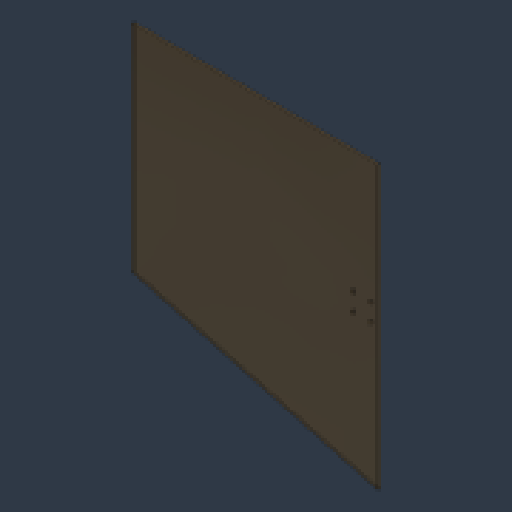
# Autodesk Inventor part: hopper_side_l
Saved by Autodesk Inventor 2024.3 (Build 283343000, 343)
## iProperties
Created: 2025-03-07
Part Number: hopper_side_l
Material: Polycarbonate, Smoke
Document SubType Name: Sheet Metal
Designer: marcu
Density: 1.2 g/cm^3
Sheet Metal Rule: Default
Appearance: Polycarbonate - Smoked
Author: marcu
Autodesk Inventor part; units mm, degrees
ref_plane "YZ Plane" through (0, 0, 0) normal (1, 0, 0) x (0, 1, 0)
ref_plane "XZ Plane" through (0, 0, 0) normal (0, 1, 0) x (-1, 0, 0)
ref_plane "XY Plane" through (0, 0, 0) normal (0, 0, 1) x (1, 0, 0)
sketch "Sketch1" plane through (0, 0, 0) normal (0, 0, 1) x (1, 0, 0)
  line L0 (-177.8, 203.2) -> (177.8, 203.2)
  line L1 (177.8, 203.2) -> (177.8, -203.2)
  line L2 (177.8, -203.2) -> (-177.8, -203.2)
  line L3 (-177.8, -203.2) -> (-177.8, 203.2)
  line L4 (-177.8, 203.2) -> (177.8, -203.2) construction
  line L5 (177.8, 203.2) -> (-177.8, -203.2) construction
  point P0 (0, 0)
  dimension "d0" = 355.6
  dimension "d1" = 406.4
  measures "d0" distance of L1.end L2.end
  measures "d1" distance of L0.end L1.end
extrude "Plate1" add sketch "Sketch1" along normal blind 3.048
sketch "Sketch2" plane through (0, 0, 0) normal (0, 0, -1) x (-1, 0, 0)
  line L0 (177.8, -203.2) -> (-177.8, -203.2) construction
  line L1 (177.8, 203.2) -> (177.8, -203.2) construction
  line L2 (-177.8, 203.2) -> (177.8, 203.2) construction
  line L3 (-177.8, -203.2) -> (-177.8, 203.2) construction
  line L4 (-177.8, -203.2) -> (177.8, -107.9173)
  line L5 (-177.8, -203.2) -> (190.3442, -203.2) construction
  line L6 (177.8, 203.2) -> (177.8, -203.2) construction
  line L7 (177.8, -107.9173) -> (177.8, -203.2)
  line L8 (177.8, -203.2) -> (-177.8, -203.2)
  point P0 (0, 0)
  dimension "d3" = 15
  constraints: 8 end point, 2 collinear, 2 point on line, 1 equal length, 1 horizontal
  measures "d3" angle of L5 L4
extrude "Cut1" cut sketch "Sketch2" against normal blind 3.048
sketch "Sketch3" plane through (0, 0, 0) normal (0, 0, -1) x (-1, 0, 0)
  line L0 (-177.8, -203.2) -> (177.8, -107.9173) construction
  line L1 (177.8, 203.2) -> (177.8, -107.9173) construction
  line L2 (-177.8, 203.2) -> (177.8, 203.2) construction
  line L3 (-177.8, -203.2) -> (-177.8, 203.2) construction
  line L4 (-177.8, 0) -> (-165.1, 0) construction
  point P0 (0, 0)
  point P1 (-139.7, 0)
  point P2 (-165.1, 25.4)
  point P3 (-139.7, 25.4)
  dimension "d6" = 12.7
  dimension "d9" = 25.4
  dimension "d12" = 25.4
  constraints: 2 end point, 2 horizontal, 1 coincident, 1 midpoint, 1 vertical, 3 other
  measures "d6" distance of L4.start L4.end
  measures "d9" distance of point (-165.1, 0) point (-139.7, 0)
  measures "d12" distance of point (-165.1, 0) point (-165.1, 25.4)
hole "Hole1" at (165.1, 0, 0) at (139.7, 0, 0) at (165.1, 25.4, 0) at (139.7, 25.4, 0) direction (0, 0, 1) diameter 5.1054 end through all clearance for "Flat Head Machine Screw (82)" size "#10" standard "Ansi Unified Screw Threads"
equation "\"d4\" = Thickness"
equation "\"d20\" = Thickness"
equation "\"d2\" = Thickness"
equation "\"BendRadius\" = Thickness"
equation "\"BendReliefWidth\" = Thickness"
equation "\"BendReliefDepth\" = 0.5 * Thickness"
equation "\"CornerReliefSize\" = 4 * Thickness"
equation "\"MinimumRemnant\" = 2 * Thickness"
equation "\"TransitionRadius\" = BendRadius"
equation "\"JacobiRadiusSize\" = BendRadius"
equation "\"GapSize\" = Thickness"
equation "\"Thickness\" = 3.048"
body "Solid1"
